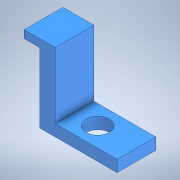
# Autodesk Inventor part: CableGuide
Saved by Autodesk Inventor 2021 (Build 250183000, 183)
## iProperties
Created: 2021-11-17
Part Number: CableGuide
Material: Generic
Document SubType Name: Modeling
Designer: Jorian Brusind
Density: 1 g/cm^3
Appearance: Cyan
Author: Jorian Brusind
Autodesk Inventor part; units mm, degrees
ref_plane "YZ Plane" through (0, 0, 0) normal (1, 0, 0) x (0, 1, 0)
ref_plane "XZ Plane" through (0, 0, 0) normal (0, 1, 0) x (-1, 0, 0)
ref_plane "XY Plane" through (0, 0, 0) normal (0, 0, 1) x (1, 0, 0)
sketch "Sketch1" plane through (0, 0, 0) normal (0, 1, 0) x (-1, 0, 0)
  line L0 (0, 0) -> (20, 0)
  line L1 (20, 0) -> (20, -10)
  line L2 (20, -10) -> (0, -10)
  line L3 (0, -10) -> (0, 0)
  dimension "d0" = 20
  dimension "d1" = 10
  constraints: 8 end point, 2 parallel, 1 horizontal, 1 perpendicular
  measures "d0" distance of L1.end L2.end
  measures "d1" distance of L0.end L1.end
extrude "Extrusion1" add sketch "Sketch1" along normal blind 3
sketch "Sketch2" plane through (0, 3, 0) normal (0, 1, 0) x (1, 0, 0)
  circle A0 centre (-10, 5) radius 3
  line L0 (0, 0) -> (0, 10) projected
  line L1 (0, 10) -> (-20, 10) projected
  dimension "d4" = 6
  dimension "d5" = 10
  dimension "d6" = 5
  constraints: 1 centre point
  measures "d4" diameter of A0
  measures "d5" distance from line of L0 A0.centre
  measures "d6" distance from line of L1 A0.centre
extrude "Extrusion2" cut sketch "Sketch2" against normal through all
sketch "Sketch3" plane through (0, 3, 0) normal (0, 1, 0) x (1, 0, 0)
  circle A0 centre (-10, 5) radius 3 projected
  circle A1 centre (-10, 5) radius 5
  line L0 (-10, 5) -> (-18, 5)
  line L1 (0, 10) -> (-20, 10) projected
  line L2 (-20, 0) -> (-16, 0)
  line L3 (-16, 0) -> (-16, 10)
  line L4 (-16, 10) -> (-20, 10)
  line L5 (-20, 10) -> (-20, 0)
  line L6 (-20, 0) -> (-16, 10) construction
  line L7 (-16, 0) -> (-20, 10) construction
  point P0 (0, 0)
  dimension "d9" = 10
  dimension "d10" = 8
  dimension "d11" = 4
  constraints: 14 end point, 2 horizontal, 2 midpoint, 2 parallel, 1 centre point, 1 coincident, 1 perpendicular, 1 point on line
  measures "d9" diameter of A1
  measures "d10" distance of L0.start L0.end
  measures "d11" distance of L4.end L3.end
extrude "Extrusion3" add sketch "Sketch3" along normal blind 17 contours L3 L2 L5 L1
sketch "Sketch4" plane through (-20, 0, -10) normal (-1, 0, 0) x (0, 0, 1)
  line L0 (0, 0) -> (0, 20) projected
  line L1 (0, 20) -> (10, 20)
  line L2 (10, 20) -> (10, 18)
  line L3 (10, 18) -> (0, 18)
  line L4 (0, 18) -> (0, 20)
  point P0 (10, 0)
  dimension "d14" = 10
  dimension "d15" = 2
  constraints: 8 end point, 2 parallel, 1 horizontal, 1 perpendicular
  measures "d14" distance of L2.end L3.end
  measures "d15" distance of L1.end L2.end
extrude "Extrusion4" add sketch "Sketch4" along normal blind 4
body "Solid1"
